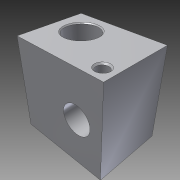
# Autodesk Inventor part: heatblock
Saved by Autodesk Inventor 2014 (Build 180170000, 170)
## iProperties
Created: 2014-03-25
Part Number: heatblock
Material: Aluminum 6061
Document SubType Name: Modeling
Designer: buben
Density: 2.71 g/cm^3
Appearance: Aluminum - Flat
Mass: 6.39589 g
Surface Area: 17.0713 cm^2
Volume: 2.36011 cm^3
Author: buben
Autodesk Inventor part; units mm, degrees
ref_plane "YZ Plane" through (0, 0, 0) normal (1, 0, 0) x (0, 1, 0)
ref_plane "XZ Plane" through (0, 0, 0) normal (0, 1, 0) x (-1, 0, 0)
ref_plane "XY Plane" through (0, 0, 0) normal (0, 0, 1) x (1, 0, 0)
sketch "Sketch1" plane through (0, 0, 0) normal (0, 1, 0) x (-1, 0, 0)
  line L0 (0, 0) -> (-16, 0)
  line L1 (-16, 0) -> (-16, -16)
  line L2 (-16, -16) -> (0, -16)
  line L3 (0, -16) -> (0, 0)
  dimension "d0" = 16
  constraints: 8 end point, 2 parallel, 2 perpendicular, 1 horizontal
  measures "d0" distance from line of L1 L2.end
extrude "Extrusion1" add sketch "Sketch1" along normal blind 12
sketch "Sketch2" plane through (16, 0, -16) normal (0, 0, -1) x (-1, 0, 0)
  line L0 (16, 0) -> (16, 12) projected
  line L1 (0, 12) -> (16, 12) projected
  circle A0 centre (11, 7.3) radius 3
  dimension "d3" = 6
  dimension "d4" = 5
  dimension "d5" = 4.7
  constraints: 1 centre point
  measures "d3" diameter of A0
  measures "d4" distance from line of A0.centre L0
  measures "d5" distance from line of A0.centre L1
extrude "Extrusion2" cut sketch "Sketch2" against normal through all
sketch "Sketch3" plane through (0, 0, 0) normal (0, 0, 1) x (1, 0, 0)
  line L0 (0, 0) -> (16, 0) projected
  line L1 (16, 0) -> (16, 12) projected
  point P0 (13.9, 2.1)
  dimension "d8" = 2.1
  dimension "d9" = 2.1
  measures "d8" distance from line of point (13.9, 2.1) L1
  measures "d9" distance from line of L0 point (13.9, 2.1)
hole "Hole1" at (13.9, 2.1, 0) direction (0, 0, -1) diameter 2 depth 5 tip angle 118 countersink diameter 2.5 countersink angle 90
sketch "Sketch4" plane through (0, 12, 0) normal (0, 1, 0) x (1, 0, 0)
  line L0 (16, 0) -> (16, 16) projected
  line L1 (0, 16) -> (0, 0) projected
  circle A0 centre (11.5, 8) radius 2.5
  point P0 (0, 8)
  dimension "d17" = 5
  dimension "d18" = 4.5
  constraints: 1 centre point, 1 horizontal alignment, 1 midpoint
  measures "d17" diameter of A0
  measures "d18" distance from line of L0 A0.centre
extrude "Extrusion3" cut sketch "Sketch4" against normal through all
sketch "Sketch5" plane through (0, 0, -16) normal (-1, 0, 0) x (0, 0, 1)
  line L0 (0, 12) -> (16, 12) projected
  line L1 (0, 4.3) -> (0, 10.3) projected
  line L2 (16, 10.3) -> (16, 4.3) projected
  line L3 (0, 4.3) -> (0, 10.3) projected
  line L4 (0, 7.3) -> (16, 7.3) construction
  circle A0 centre (8, 7.3) radius 1
  dimension "d21" = 4.7
  dimension "d22" = 2
  constraints: 3 midpoint, 2 end point, 1 centre point, 1 perpendicular
  measures "d21" distance between parallel lines of L0 L4
  measures "d22" diameter of A0
extrude "Extrusion4" cut sketch "Sketch5" against normal up to surface
thread "Thread1" size "M2x0.4" class "6H" standard "ANSI Metric M Profile" full length
chamfer "Chamfer1" distance 0.2 angle 45 1 edges at (0, 7.3, -9)
chamfer "Chamfer2" distance 0.2 angle 45 2 edges at (8, 7.3, 0) (8, 7.3, -16)
equation "\"d9\" = d8"
body "Solid1"
